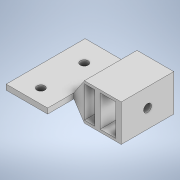
# Autodesk Inventor part: VbearingBracket
Saved by Autodesk Inventor 2020 (Build 240168000, 168)
## iProperties
Created: 2020-01-12
Part Number: VbearingBracket
Material: Generic
Document SubType Name: Modeling
Designer: tdmp4
Density: 1 g/cm^3
Appearance: Default
Author: tdmp4
Autodesk Inventor part; units mm, degrees
ref_plane "YZ Plane" through (0, 0, 0) normal (1, 0, 0) x (0, 1, 0)
ref_plane "XZ Plane" through (0, 0, 0) normal (0, 1, 0) x (-1, 0, 0)
ref_plane "XY Plane" through (0, 0, 0) normal (0, 0, 1) x (1, 0, 0)
sketch "Sketch1" plane through (0, 0, 0) normal (0, 1, 0) x (-1, 0, 0)
  line L0 (0, -27.8975) -> (20, -27.8975)
  line L1 (20, -27.8975) -> (20, -53.2975)
  line L2 (20, -53.2975) -> (0, -53.2975)
  line L3 (0, -53.2975) -> (0, -27.8975)
  point P0 (0, 0)
  dimension "d0" = 20
  dimension "d1" = 25.4
  constraints: 8 end point, 2 parallel, 1 horizontal, 1 perpendicular
  measures "d0" distance of L1.end L2.end
  measures "d1" distance of L2.end L0.start
extrude "Extrusion1" add sketch "Sketch1" along normal blind 2.54
sketch "Sketch2" plane through (0, 0, -27.8975) normal (1, 0, 0) x (0, 0, -1)
  line L0 (0, 0) -> (25.4, 0) projected
  line L1 (0, 2.54) -> (25.4, 2.54)
  line L2 (25.4, 2.54) -> (25.4, 0)
  line L3 (25.4, 0) -> (0, 0)
  line L4 (0, 0) -> (0, 2.54)
  point P0 (-27.8975, 0)
  constraints: 8 end point, 2 parallel, 1 horizontal, 1 perpendicular
extrude "Extrusion2" add sketch "Sketch2" along normal blind 5.08
sketch "Sketch4" plane through (-20, 0, -27.8975) normal (0, 0, 1) x (1, 0, 0)
  line L0 (25.08, 2.54) -> (25.08, 0) construction
  line L1 (25.08, 2.54) -> (20, 2.54) construction
  line L2 (0, 0) -> (25.08, 0) projected
  line L3 (25.08, 0) -> (20, 0)
  line L4 (0, 2.54) -> (25.08, 2.54) projected
  line L5 (25.08, 2.54) -> (25.08, 10.16)
  line L6 (25.08, 0) -> (25.08, -7.62)
  line L7 (20, 2.54) -> (25.08, 10.16)
  line L8 (20, 0) -> (25.08, -7.62)
  line L9 (25.08, 10.16) -> (40.32, 10.16)
  line L10 (40.32, 10.16) -> (40.32, 7.628)
  line L11 (25.08, 8.898) -> (25.08, 10.16)
  line L12 (25.08, -7.62) -> (40.32, -7.62)
  line L13 (40.32, -7.62) -> (40.32, -7.6153)
  line L14 (25.08, -7.6153) -> (25.08, -7.62)
  line L15 (40.32, 10.16) -> (42.8586, 10.16)
  line L16 (42.8586, 10.16) -> (42.8586, -7.62)
  line L17 (42.8586, -7.62) -> (40.32, -7.62)
  line L18 (40.32, -7.62) -> (40.32, 10.16)
  line L19 (40.32, -7.6177) -> (25.08, -7.6177)
  line L20 (40.32, -7.6177) -> (25.08, -7.6177)
  line L21 (25.08, -7.6177) -> (25.08, -6.3417)
  line L22 (25.08, -6.3417) -> (40.32, -6.3417)
  line L23 (40.32, -6.3417) -> (40.32, -7.6177)
  line L24 (40.32, 10.16) -> (25.08, 10.16)
  line L25 (25.08, 10.16) -> (25.08, 8.898)
  line L26 (25.08, 8.898) -> (40.32, 8.898)
  line L27 (40.32, 8.898) -> (40.32, 10.16)
  line L28 (32.7, 8.898) -> (30.1596, 8.898)
  line L29 (30.1596, 8.898) -> (30.1596, -6.3417)
  line L30 (30.1596, -6.3417) -> (32.7, -6.3417)
  line L31 (32.7, -6.3417) -> (32.7, 8.898)
  dimension "d6" = 7.62
  dimension "d7" = 2.54
  dimension "d9" = 7.62
  dimension "d10" = 15.24
  dimension "d16" = 15.24
  dimension "d30" = 17.78
  constraints: 58 end point, 10 parallel, 8 horizontal, 7 perpendicular, 4 point on line, 2 midpoint, 1 vertical
  measures "d6" distance of L0.start L5.end
  measures "d7" distance of L0.start L0.end
  measures "d9" distance of L0.end L6.end
  measures "d10" distance of L5.end L9.end
  measures "d16" distance of L13.end L14.start
  measures "d30" distance of L15.end L16.end
extrude "Extrusion3" add sketch "Sketch4" against normal blind 25.4 contours L2 L6 L8 | L6 L22 L18 L13 L19 | L13 L18 L10 L15 L16 L17 | L29 L26 L31 L22 | L26 L5 L9 L10 | L5 L4 L7
sketch "Sketch6" plane through (22.8586, -7.62, -27.8975) normal (1, 0, 0) x (0, 0, -1)
  line L0 (25.4, 10.16) -> (25.4, 17.78) projected
  line L1 (0, 7.62) -> (0, 0) projected
  line L2 (25.4, 17.78) -> (0, 17.78)
  line L3 (0, 17.78) -> (0, 0)
  line L4 (0, 0) -> (25.4, 0)
  line L5 (25.4, 0) -> (25.4, 17.78)
  line L6 (0, 17.78) -> (0, 10.16) projected
  line L7 (25.4, 0) -> (0, 17.78)
  line L8 (0, 0) -> (25.4, 17.78)
  circle A0 centre (12.7, 8.89) radius 1.905
  point P0 (-27.8975, 7.62)
  dimension "d17" = 3.81
  constraints: 12 end point, 2 parallel, 1 centre point, 1 horizontal, 1 midpoint, 1 perpendicular
  measures "d17" diameter of A0
extrude "Extrusion5" cut sketch "Sketch6" against normal blind 14.2875 contours A0 L7 L8 | L8 L7 A0 | A0 L8 L7 | L7 L8 A0
sketch "Sketch7" plane through (0, 2.54, 0) normal (0, 1, 0) x (1, 0, 0)
  line L0 (-20, 27.8975) -> (0, 27.8975) projected
  line L1 (0, 27.8975) -> (0, 53.2975) projected
  line L2 (-20, 27.8975) -> (0, 27.8975)
  line L3 (0, 27.8975) -> (0, 42.8975)
  line L4 (0, 42.8975) -> (-20, 42.8975)
  line L5 (-20, 42.8975) -> (-20, 27.8975)
  circle A0 centre (-10, 42.8975) radius 1.905
  point P0 (0, 0)
  dimension "d20" = 15
  dimension "d21" = 3.81
  constraints: 8 end point, 2 parallel, 1 centre point, 1 horizontal, 1 midpoint, 1 perpendicular, 1 point on line
  measures "d20" distance of L4.end L0.start
  measures "d21" diameter of A0
extrude "Extrusion6" cut sketch "Sketch7" against normal blind 28.575 contours A0 L4 | L4 A0
sketch "Sketch8" plane through (-20, 0, -27.8975) normal (0, 0, 1) x (1, 0, 0)
  line L0 (0, 0) -> (20, 0) projected
  line L1 (0, 2.54) -> (20, 2.54) projected
  line L2 (0, 0) -> (20, 0)
  line L3 (20, 0) -> (20, 2.54)
  line L4 (20, 2.54) -> (0, 2.54)
  line L5 (0, 2.54) -> (0, 0)
  constraints: 8 end point, 2 parallel, 1 horizontal, 1 perpendicular
extrude "Extrusion7" add sketch "Sketch8" along normal blind 12.7
sketch "Sketch9" plane through (0, 2.54, 0) normal (0, 1, 0) x (1, 0, 0)
  circle A0 centre (-10, 21.9147) radius 1.905
  point P0 (0, 0)
  dimension "d26" = 3.81
  constraints: 1 centre point
  measures "d26" diameter of A0
extrude "Extrusion8" cut sketch "Sketch9" against normal blind 76.2
body "Solid1"
